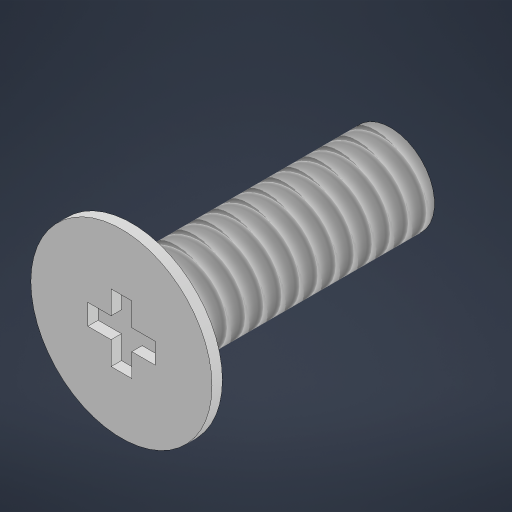
# Autodesk Inventor part: M1.7x5
Saved by Autodesk Inventor 2024.2 (Build 282272000, 272)
## iProperties
Created: 2024-01-06
Part Number: M1.7x5
Material: 一般
Document SubType Name: Modeling
Designer: Hanaoka
Density: 1 g/cm^3
Appearance: 既定
Author: Hanaoka
Autodesk Inventor part; units mm, degrees
ref_plane "YZ Plane" through (0, 0, 0) normal (1, 0, 0) x (0, 1, 0)
ref_plane "XZ Plane" through (0, 0, 0) normal (0, 1, 0) x (-1, 0, 0)
ref_plane "XY Plane" through (0, 0, 0) normal (0, 0, 1) x (1, 0, 0)
sketch "スケッチ1" plane through (0, 0, 0) normal (0, 0, 1) x (1, 0, 0)
  circle A0 centre (0, 0) radius 1.75
  line L0 (0.2, -0.65) -> (-0.2, -0.65)
  line L1 (-0.2, -0.65) -> (-0.2, 0.65)
  line L2 (-0.2, 0.65) -> (0.2, 0.65)
  line L3 (0.2, 0.65) -> (0.2, -0.65)
  line L4 (0.2, -0.65) -> (-0.2, 0.65) construction
  line L5 (-0.2, -0.65) -> (0.2, 0.65) construction
  line L6 (0.65, -0.2) -> (-0.65, -0.2)
  line L7 (-0.65, -0.2) -> (-0.65, 0.2)
  line L8 (-0.65, 0.2) -> (0.65, 0.2)
  line L9 (0.65, 0.2) -> (0.65, -0.2)
  line L10 (0.65, -0.2) -> (-0.65, 0.2) construction
  line L11 (-0.65, -0.2) -> (0.65, 0.2) construction
  point P0 (-0.2, -0.2)
  point P1 (-0.2, 0.2)
  point P2 (0.2, 0.2)
  point P3 (0.2, -0.2)
  dimension "d0" = 3.5
  dimension "d1" = 0.4
  dimension "d2" = 1.3
  constraints: 24 end point, 4 midpoint, 4 parallel, 4 perpendicular, 2 horizontal, 1 centre point, 1 coincident
  measures "d0" diameter of A0
  measures "d1" distance of L8.end L6.start
  measures "d2" distance of L2.end L0.start
extrude "押し出し1" add sketch "スケッチ1" along normal blind 0.2
sketch "スケッチ2" plane through (0, 0, 0) normal (0, 0, -1) x (-1, 0, 0)
  circle A0 centre (0, 0) radius 0.85
  dimension "d5" = 1.7
  constraints: 1 centre point, 1 coincident
  measures "d5" diameter of A0
extrude "押し出し2" add sketch "スケッチ2" along normal blind 5
thread "ねじ1" size "M1.7x0.35" class "6g" standard "ANSI Metric M Profile" full length
